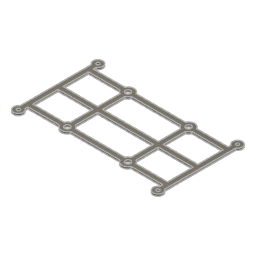
fc_vibration_dumper_DJI_F450 (Autodesk Fusion 360 design; units mm, degrees)
Autodesk Fusion 360 part; units mm, degrees
sketch "Sketch1" plane through (0, 0, 0) normal (0, 1, 0) x (1, 0, 0) in component "vibration_dumper_part_1"
  line L0 (0, 0) -> (62.5, 0)
  line L1 (62.5, 0) -> (62.5, -39.5)
  line L2 (62.5, -39.5) -> (0, -39.5)
  line L3 (0, -39.5) -> (0, 0)
  circle A0 centre (0, 0) radius 1.6
  circle A1 centre (62.5, 0) radius 1.6
  circle A2 centre (62.5, -39.5) radius 1.6
  circle A3 centre (0, -39.5) radius 1.6
  line L4 (0, -39.5) -> (0, -37)
  line L5 (62.5, -39.5) -> (62.5, -41.1)
  line L6 (62.5, -39.5) -> (62.5, -42)
  line L7 (0, -37) -> (62.5, -37)
  line L8 (62.5, -37) -> (62.5, -42)
  line L9 (62.5, -42) -> (0, -42)
  line L10 (0, -42) -> (0, -37)
  line L11 (0, -39.5) -> (2.5, -39.5)
  line L12 (0, 0) -> (-2.5, 0)
  line L13 (-2.5, 0) -> (2.5, 0)
  line L14 (2.5, 0) -> (2.5, -39.5)
  line L15 (2.5, -39.5) -> (-2.5, -39.5)
  line L16 (-2.5, -39.5) -> (-2.5, 0)
  line L17 (62.5, 0) -> (62.5, 2.5)
  line L18 (62.5, 2.5) -> (0, 2.5)
  line L19 (0, 2.5) -> (0, -2.5)
  line L20 (0, -2.5) -> (62.5, -2.5)
  line L21 (62.5, -2.5) -> (62.5, 2.5)
  line L22 (62.5, -39.5) -> (65, -39.5)
  line L23 (65, -39.5) -> (60, -39.5)
  line L24 (60, -39.5) -> (60, 0)
  line L25 (60, 0) -> (65, 0)
  line L26 (65, 0) -> (65, -39.5)
  circle A4 centre (0, 0) radius 5
  circle A5 centre (62.5, 0) radius 5
  circle A6 centre (0, -39.5) radius 5
  circle A7 centre (62.5, -39.5) radius 5
  line L27 (0, -39.5) -> (0, -51)
  line L28 (0, 0) -> (0, 11.5)
  line L29 (0, 11.5) -> (62.5, 11.5)
  line L30 (62.5, 11.5) -> (62.5, -51)
  line L31 (62.5, -51) -> (0, -51)
  line L32 (0, -51) -> (0, 11.5)
  circle A8 centre (0, 11.5) radius 2.75
  circle A9 centre (62.5, 11.5) radius 2.75
  circle A10 centre (0, -51) radius 2.75
  circle A11 centre (62.5, -51) radius 2.75
  circle A12 centre (0, 11.5) radius 6.25
  circle A13 centre (0, -51) radius 6.25
  circle A14 centre (62.5, -51) radius 6.25
  circle A15 centre (62.5, 11.5) radius 6.25
  line L33 (60, 0) -> (65, 0)
  line L34 (65, 0) -> (65, 7)
  line L35 (65, 7) -> (60, 7)
  line L36 (60, 7) -> (60, 0)
  line L37 (-2.5, 0) -> (2.5, 0)
  line L38 (2.5, 0) -> (2.5, 7)
  line L39 (2.5, 7) -> (-2.5, 7)
  line L40 (-2.5, 7) -> (-2.5, 0)
  line L41 (-2.5, -39.5) -> (2.5, -39.5)
  line L42 (2.5, -39.5) -> (2.5, -46.5)
  line L43 (2.5, -46.5) -> (-2.5, -46.5)
  line L44 (-2.5, -46.5) -> (-2.5, -39.5)
  line L45 (60, -39.5) -> (65, -39.5)
  line L46 (65, -39.5) -> (65, -46.5)
  line L47 (65, -46.5) -> (60, -46.5)
  line L48 (60, -46.5) -> (60, -39.5)
  dimension "d1" = 62.5
  dimension "d2" = 39.5
  dimension "d3" = 3.2
  dimension "d4" = 3.2
  dimension "d5" = 3.2
  dimension "d6" = 3.2
  dimension "d7" = 2.5
  dimension "d8" = 2.5
  dimension "d9" = 2.5
  dimension "d10" = 5
  dimension "d11" = 5
  dimension "d12" = 10
  dimension "d13" = 10
  dimension "d14" = 10
  dimension "d15" = 10
  dimension "d18" = 11.5
  dimension "d19" = 11.5
  dimension "d20" = 62.5
  dimension "d21" = 5.5
  dimension "d22" = 5.5
  dimension "d23" = 5.5
  dimension "d24" = 5.5
  dimension "d25" = 12.5
  dimension "d26" = 12.5
  dimension "d27" = 12.5
  dimension "d28" = 12.5
  dimension "d29" = 7
  dimension "d30" = 7
  dimension "d31" = 7
  constraint horizontal L0
  constraint vertical L1
  constraint horizontal L2
  constraint vertical L3
  constraint coincident L0.start L3.end
  constraint coincident L0.end L1.start
  constraint coincident L1.end L2.start
  constraint coincident L2.end L3.start
  constraint perpendicular L2 L4
  constraint coincident A2 L5.end
  constraint perpendicular L2 L5
  constraint parallel L5 L6
  constraint horizontal L7
  constraint vertical L8
  constraint horizontal L9
  constraint vertical L10
  constraint perpendicular L4 L11
  constraint perpendicular L3 L12
  constraint horizontal L13
  constraint vertical L14
  constraint horizontal L15
  constraint vertical L16
  constraint perpendicular L0 L17
  constraint horizontal L18
  constraint vertical L19
  constraint horizontal L20
  constraint vertical L21
  constraint coincident L3 L19.end
  constraint perpendicular L5 L22
  constraint horizontal L23
  constraint vertical L24
  constraint horizontal L25
  constraint vertical L26
  constraint coincident L0 L24.end
  constraint concentric A1 A5
  constraint concentric A3 A6
  constraint perpendicular L15 L27
  constraint perpendicular L0 L28
  constraint horizontal L29
  constraint vertical L30
  constraint horizontal L31
  constraint vertical L32
  constraint coincident L28.end L29.start
  constraint coincident L29.end L30.start
  constraint coincident L27.end L31.end
  constraint coincident L30.end L31.start
  constraint concentric A8 A12
  constraint concentric A11 A14
  constraint concentric A9 A15
  constraint horizontal L33
  constraint vertical L34
  constraint horizontal L35
  constraint vertical L36
  constraint horizontal L37
  constraint vertical L38
  constraint horizontal L39
  constraint vertical L40
  constraint horizontal L41
  constraint vertical L42
  constraint horizontal L43
  constraint vertical L44
  constraint horizontal L45
  constraint vertical L46
  constraint horizontal L47
  constraint vertical L48
  measures "d1" distance of L0.start L0.end
  measures "d2" distance of L0.start L2.end
  measures "d3" diameter of A0
  measures "d4" diameter of A1
  measures "d5" diameter of A2
  measures "d6" diameter of A3
  measures "d7" distance of L2.end L4.end
  measures "d8" distance of L1.end L6.end
  measures "d9" distance of L2.end L11.end
  measures "d10" distance of L17.end L20.end
  measures "d11" distance of L22.end L23.end
  measures "d12" diameter of A4
  measures "d13" diameter of A5
  measures "d14" diameter of A6
  measures "d15" diameter of A7
  measures "d18" distance of L2.end L27.end
  measures "d19" distance of L0.start L28.end
  measures "d20" distance of L28.end L27.end
  measures "d21" diameter of A8
  measures "d22" diameter of A9
  measures "d23" diameter of A10
  measures "d24" diameter of A11
  measures "d25" diameter of A12
  measures "d26" diameter of A13
  measures "d27" diameter of A14
  measures "d28" diameter of A15
  measures "d29" distance of L12.end L39.end
  measures "d30" distance of L15.end L43.end
  measures "d31" distance of L23.end L47.end
extrude "Extrude1" add sketch "Sketch1" along normal blind 2 contours L0 A0 L13 L18 L19 L28 L32 L37 L38 | L0 L3 A0 L13 L14 L19 L20 L32 L37 | L3 A0 L12 L13 L16 L19 A4 L32 L37 | A0 L12 L13 L19 A4 L28 L32 L37 L40 | L0 L18 A4 L38 | L0 L14 L20 A4 | L3 L14 L20 A4 L32 | L16 A4 L40 | L18 A4 L28 L32 L38 | L0 L18 A4 A5 | L0 L20 A4 A5 | L14 L20 A4 | L18 A4 L38 | L3 L14 A4 A6 L32 | L3 L16 A4 A6 L32 | L0 L18 A5 L36 | L0 L20 L24 A5 | L3 L7 L14 A6 L32 | L3 A3 L4 L10 L15 L16 A6 L32 L41 | L16 A6 L44 | L0 A1 L17 L18 L21 L25 L30 L33 L36 | L0 L1 A1 L20 L21 L24 L25 L30 L33 | L18 A5 L36 | L20 L24 A5 | L7 L14 A6 | L2 L3 A3 L4 L7 L10 L11 L14 L15 L32 L41 | A3 L10 L15 A6 L27 L32 L41 L44 | L1 L20 L24 A5 L30 | L18 A5 L30 L36 | L1 L24 A5 A7 L30 | L2 L7 L14 A6 | L2 L7 A6 A7 | L9 A6 L27 L32 L42 | A1 L17 L21 L25 A5 L30 L33 L34 | L1 A1 L21 L25 L26 A5 L30 L33 | L1 L7 L24 A7 L30 | L7 L24 A7 | L1 L26 A5 A7 L30 | L2 A3 L9 L10 L11 L15 L27 L32 L41 L42 | L2 L9 A6 L42 | L2 L7 L24 A7 | L2 L9 A6 A7 | L9 A6 L42 | L26 A5 L34 | L1 L2 A2 L7 L8 L23 L24 L30 L45 | L1 A2 L8 L22 L23 L26 A7 L30 L45 | L2 L9 A7 L48 | L2 A2 L6 L8 L9 L23 L30 L45 L48 | L26 A7 L46 | L9 A7 L48 | L9 A7 L30 L48 | A2 L6 L8 L22 L23 A7 L30 L45 L46 makes body 1 in component "vibration_dumper_part_1"
extrude "Extrude2" add sketch "Sketch1" along normal blind 2 contours A4 L28 L32 A12 L40 | A4 L28 L32 A12 L38 | L28 L32 A12 L39 L40 | L28 L29 L32 A8 A12 L39 L40 | L28 L32 A12 L38 L39 | L28 L29 L32 A8 A12 L38 L39 | A6 L27 L32 A13 L44 | A5 L30 A15 L36 | A6 L27 L32 A13 L42 | L27 L31 L32 A10 A13 L43 L44 | L27 L32 A13 L43 L44 | L29 L30 A9 A15 L34 L35 | L29 L30 A9 A15 L35 L36 | A5 L30 A15 L34 | L30 A15 L35 L36 | L27 L32 A13 L42 L43 | L27 L31 L32 A10 A13 L42 L43 | L30 A15 L34 L35 | L30 L31 A11 A14 L47 L48 | L30 L31 A11 A14 L46 L47 | A7 L30 A14 L48 | L30 A14 L47 L48 | L30 A14 L46 L47 | A7 L30 A14 L46 bodies 1 in component "vibration_dumper_part_1"
sketch "Sketch2" plane through (0, 0, 0) normal (0, 1, 0) x (1, 0, 0) in component "vibration_dumper_part_1"
  circle A0 centre (62.5, 11.5) radius 2.75
  circle A1 centre (62.5, 11.5) radius 6.25
  circle A2 centre (0, 11.5) radius 2.75
  circle A3 centre (0, 11.5) radius 6.25
  circle A4 centre (0, -51) radius 2.75
  circle A5 centre (0, -51) radius 6.25
  circle A6 centre (62.5, -51) radius 2.6926
  circle A7 centre (62.5, -51) radius 6.25
  line L0 (65, -46.5) -> (60, -46.5)
  line L1 (60, -46.5) -> (60, 7)
  line L2 (60, 7) -> (65, 7)
  line L3 (65, 7) -> (65, -46.5)
  line L4 (2.5, -46.5) -> (-2.5, -46.5)
  line L5 (-2.5, -46.5) -> (-2.5, 7)
  line L6 (-2.5, 7) -> (2.5, 7)
  line L7 (2.5, 7) -> (2.5, -46.5)
  line L8 (62.5, 11.5) -> (62.5, -51)
  line L9 (62.5, -51) -> (62.5, -48.5)
  line L10 (0, 11.5) -> (62.5, 11.5)
  line L11 (62.5, 11.5) -> (62.5, 9)
  line L12 (62.5, 9) -> (0, 9)
  line L13 (0, 9) -> (0, 14)
  line L14 (0, 14) -> (62.5, 14)
  line L15 (62.5, 14) -> (62.5, 9)
  line L16 (62.5, -48.5) -> (0, -48.5)
  line L17 (0, -48.5) -> (0, -53.5)
  line L18 (0, -53.5) -> (62.5, -53.5)
  line L19 (62.5, -53.5) -> (62.5, -48.5)
  point P0 (62.5, 11.5)
  point P1 (0, 11.5)
  point P2 (0, -51)
  point P3 (62.5, -51)
  point P4 (65, -46.5)
  point P5 (60, 7)
  point P6 (2.5, -46.5)
  point P7 (-2.5, 7)
  dimension "d34" = 2.5
  dimension "d35" = 2.5
  dimension "d36" = 5
  dimension "d37" = 5
  constraint coincident P0 A0.centre
  constraint coincident P1 A2.centre
  constraint coincident P2 A4.centre
  constraint coincident P3 A6.centre
  constraint horizontal L0
  constraint vertical L1
  constraint horizontal L2
  constraint vertical L3
  constraint coincident P5 L1.end
  constraint coincident P4 L0.start
  constraint horizontal L4
  constraint vertical L5
  constraint horizontal L6
  constraint vertical L7
  constraint coincident P7 L5.end
  constraint coincident P6 L4.start
  constraint parallel L8 L9
  constraint perpendicular L10 L11
  constraint horizontal L12
  constraint vertical L13
  constraint horizontal L14
  constraint vertical L15
  constraint horizontal L16
  constraint vertical L17
  constraint horizontal L18
  constraint vertical L19
  measures "d34" distance of P3 L9.end
  measures "d35" distance of P0 L11.end
  measures "d36" distance of L11.end L14.end
  measures "d37" distance of L9.end L18.end
extrude "Extrude3" add sketch "Sketch2" along normal blind 2 separate body contours A0 A1 L2 L3 L8 L14 | A0 A1 L10 L14 | A0 A1 L1 L2 L8 L12 | A0 A1 L10 L12 | A1 A3 L10 L14 | A1 L1 L2 L8 | A1 L2 L3 L8 | A1 A3 L10 L12 | A2 A3 L5 L6 L7 L12 L14 | A2 A3 L10 L14 | A1 A7 L1 L8 | A1 A7 L3 L8 | A2 A3 L10 L12 | A3 L5 L6 L7 | A3 A5 L5 L7 | A7 L0 L1 L8 | A7 L0 L3 L8 | A6 A7 L0 L3 L8 L18 | A4 A5 L4 L5 L7 L16 L18 | A5 L4 L5 L7 | A6 A7 L0 L1 L8 L16 | A4 A5 L16 L18 | A5 A7 L16 L18 | A6 A7 L16 L18 makes body 2 in component "vibration_dumper_part_1"
sketch "Sketch3" plane through (0, 0, 0) normal (0, 1, 0) x (1, 0, 0) in component "vibration_dumper_part_1"
  line L0 (0, -48.5) -> (0, -53.5)
  line L1 (0, -51) -> (-43.75, -51)
  line L2 (62.5, -53.5) -> (62.5, -48.5)
  line L3 (62.5, -51) -> (106.25, -51)
  line L4 (106.25, -51) -> (103.25, -51)
  line L5 (-43.75, -51) -> (-40.75, -51)
  line L6 (103.25, 11.5) -> (-40.75, 11.5)
  line L7 (62.5, -51) -> (62.5, -64.75)
  line L8 (62.5, 11.5) -> (62.5, 25.25)
  line L9 (62.5, -64.75) -> (62.5, -60.75)
  line L10 (62.5, 25.25) -> (62.5, 21.25)
  line L11 (62.5, 21.25) -> (103.25, 21.25)
  line L12 (103.25, 21.25) -> (103.25, 11.5)
  line L13 (103.25, 11.5) -> (62.5, 11.5)
  line L14 (62.5, 11.5) -> (62.5, 21.25)
  line L15 (103.25, -51) -> (62.5, -51)
  line L16 (62.5, -51) -> (62.5, -60.75)
  line L17 (62.5, -60.75) -> (103.25, -60.75)
  line L18 (103.25, -60.75) -> (103.25, -51)
  line L19 (0, -51) -> (-40.75, -51)
  line L20 (-40.75, -51) -> (-40.75, -60.75)
  line L21 (-40.75, -60.75) -> (0, -60.75)
  line L22 (0, -60.75) -> (0, -51)
  line L23 (0, 11.5) -> (-40.75, 11.5)
  line L24 (-40.75, 11.5) -> (-40.75, 21.25)
  line L25 (-40.75, 21.25) -> (0, 21.25)
  line L26 (0, 21.25) -> (0, 11.5)
  circle A0 centre (103.25, -60.75) radius 1.6
  circle A1 centre (103.25, -60.75) radius 5
  circle A2 centre (-40.75, -60.75) radius 1.6
  circle A3 centre (-40.75, -60.75) radius 5
  circle A4 centre (-40.75, 21.25) radius 1.6
  circle A5 centre (-40.75, 21.25) radius 5
  circle A6 centre (103.25, 21.25) radius 1.6
  circle A7 centre (103.25, 21.25) radius 5
  line L27 (103.25, -60.75) -> (105.75, -60.75)
  line L28 (105.75, -60.75) -> (100.75, -60.75)
  line L29 (100.75, -60.75) -> (100.75, 21.25)
  line L30 (100.75, 21.25) -> (105.75, 21.25)
  line L31 (105.75, 21.25) -> (105.75, -60.75)
  line L32 (-40.75, -60.75) -> (-43.25, -60.75)
  line L33 (-43.25, -60.75) -> (-38.25, -60.75)
  line L34 (-38.25, -60.75) -> (-38.25, 21.25)
  line L35 (-38.25, 21.25) -> (-43.25, 21.25)
  line L36 (-43.25, 21.25) -> (-43.25, -60.75)
  line L37 (0, 9) -> (-38.25, 9)
  line L38 (-38.25, 9) -> (-38.25, 14)
  line L39 (-38.25, 14) -> (0, 14)
  line L40 (0, 14) -> (0, 9)
  line L41 (62.5, 14) -> (100.75, 14)
  line L42 (100.75, 14) -> (100.75, 9)
  line L43 (100.75, 9) -> (62.5, 9)
  line L44 (62.5, 9) -> (62.5, 14)
  line L45 (62.5, -48.5) -> (100.75, -48.5)
  line L46 (100.75, -48.5) -> (100.75, -53.5)
  line L47 (100.75, -53.5) -> (62.5, -53.5)
  line L48 (62.5, -53.5) -> (62.5, -48.5)
  line L49 (0, -53.5) -> (-38.25, -53.5)
  line L50 (-38.25, -53.5) -> (-38.25, -48.5)
  line L51 (-38.25, -48.5) -> (0, -48.5)
  line L52 (0, -48.5) -> (0, -53.5)
  line L53 (100.75, -19.75) -> (-38.25, -19.75)
  line L54 (100.75, -19.75) -> (-38.25, -19.75)
  line L55 (-38.25, -19.75) -> (-38.25, -22.25)
  line L56 (-38.25, -22.25) -> (100.75, -22.25)
  line L57 (100.75, -22.25) -> (100.75, -19.75)
  line L58 (100.75, -19.75) -> (-38.25, -19.75)
  line L59 (-38.25, -19.75) -> (-38.25, -17.25)
  line L60 (-38.25, -17.25) -> (100.75, -17.25)
  line L61 (100.75, -17.25) -> (100.75, -19.75)
  point P0 (0, -51)
  point P1 (62.5, -51)
  point P2 (62.5, 11.5)
  point P3 (0, 11.5)
  point P4 (0, 9)
  point P5 (62.5, 14)
  dimension "d40" = 43.75
  dimension "d41" = 43.75
  dimension "d42" = 3
  dimension "d43" = 3
  dimension "d44" = 13.75
  dimension "d45" = 13.75
  dimension "d46" = 4
  dimension "d47" = 4
  dimension "d48" = 3.2
  dimension "d49" = 10
  dimension "d50" = 3.2
  dimension "d51" = 10
  dimension "d52" = 3.2
  dimension "d53" = 10
  dimension "d54" = 3.2
  dimension "d55" = 10
  dimension "d58" = 2.5
  dimension "d59" = 5
  dimension "d60" = 2.5
  dimension "d61" = 5
  dimension "d62" = 5
  dimension "d63" = 5
  dimension "d74" = 2.5
  dimension "d75" = 2.5
  constraint coincident P0 L1.start
  constraint perpendicular L0 L1
  constraint coincident P1 L3.start
  constraint perpendicular L2 L3
  constraint parallel L3 L4
  constraint parallel L1 L5
  constraint parallel L1 L6
  constraint perpendicular L3 L7
  constraint coincident P2 L8.start
  constraint perpendicular L6 L8
  constraint parallel L7 L9
  constraint parallel L8 L10
  constraint horizontal L11
  constraint vertical L12
  constraint horizontal L13
  constraint vertical L14
  constraint horizontal L15
  constraint vertical L16
  constraint horizontal L17
  constraint vertical L18
  constraint horizontal L19
  constraint vertical L20
  constraint horizontal L21
  constraint vertical L22
  constraint horizontal L23
  constraint vertical L24
  constraint horizontal L25
  constraint vertical L26
  constraint coincident P3 L23.start
  constraint coincident L17.end L18.start
  constraint concentric A0 A1
  constraint coincident L20.end L21.start
  constraint coincident L24.end L25.start
  constraint concentric A4 A5
  constraint coincident L11.end L12.start
  constraint concentric A6 A7
  constraint perpendicular L18 L27
  constraint horizontal L28
  constraint vertical L29
  constraint horizontal L30
  constraint vertical L31
  constraint perpendicular L20 L32
  constraint horizontal L33
  constraint vertical L34
  constraint horizontal L35
  constraint vertical L36
  constraint coincident L25 L34.end
  constraint horizontal L37
  constraint vertical L38
  constraint horizontal L39
  constraint vertical L40
  constraint coincident L34 L38.end
  constraint coincident P4 L37.start
  constraint horizontal L41
  constraint vertical L42
  constraint horizontal L43
  constraint vertical L44
  constraint coincident L29 L42.end
  constraint coincident P5 L41.start
  constraint horizontal L45
  constraint vertical L46
  constraint horizontal L47
  constraint vertical L48
  constraint coincident L29 L46.end
  constraint coincident L2.end L45.start
  constraint horizontal L49
  constraint vertical L50
  constraint horizontal L51
  constraint vertical L52
  constraint coincident L34 L50.end
  constraint coincident L0.end L49.start
  constraint midpoint L29 L53.start
  constraint midpoint L34 L53.end
  constraint horizontal L54
  constraint vertical L55
  constraint horizontal L56
  constraint vertical L57
  constraint horizontal L58
  constraint vertical L59
  constraint horizontal L60
  constraint vertical L61
  measures "d40" distance of P0 L1.end
  measures "d41" distance of P1 L3.end
  measures "d42" distance of L3.end L4.end
  measures "d43" distance of L1.end L5.end
  measures "d44" distance of P1 L7.end
  measures "d45" distance of P2 L8.end
  measures "d46" distance of L7.end L9.end
  measures "d47" distance of L8.end L10.end
  measures "d48" diameter of A0
  measures "d49" diameter of A1
  measures "d50" diameter of A2
  measures "d51" diameter of A3
  measures "d52" diameter of A4
  measures "d53" diameter of A5
  measures "d54" diameter of A6
  measures "d55" diameter of A7
  measures "d58" distance of L17.end L27.end
  measures "d59" distance of L27.end L28.end
  measures "d60" distance of L20.end L32.end
  measures "d61" distance of L32.end L33.end
  measures "d62" distance of P4 L39.end
  measures "d63" distance of L2.end L2.start
  measures "d74" distance of L53.start L56.end
  measures "d75" distance of L53.start L60.end
extrude "Extrude4" add sketch "Sketch3" along normal blind 2 separate body contours L21 A2 A3 L32 L33 L36 | L21 A3 L34 | L20 L21 A2 A3 L33 L34 | L20 A2 A3 L32 L33 L36 | L24 A4 A5 L35 L36 | L25 A4 A5 L35 L36 | L25 A5 L34 | L24 L25 A4 A5 L34 L35 | L18 A0 A1 L27 L28 L31 | L17 L18 A0 A1 L28 L29 | L17 A1 L29 | L11 A6 A7 L30 L31 | L12 A6 A7 L30 L31 | L17 A0 A1 L27 L28 L31 | L11 L12 A6 A7 L29 L30 | L11 A7 L29 makes body 3 at (107.0981, 0, -21.0016) makes body 4 at (-36.9079, 0, -20.9221) makes body 5 at (107.0981, 0, 60.9984) makes body 6 at (-36.9079, 0, 61.0779) in component "vibration_dumper_part_1"
extrude "Extrude5" cut sketch "Sketch3" along normal blind 2 contours L1 L5 L6 L19 L23 L24 A5 L34 L36 L38 L50 L55 L59 | L1 L19 L20 A3 L34 L50 | L1 L5 L20 A3 L36 | L3 L4 L6 L12 L13 L15 A7 L29 L31 L42 L46 L57 L61 | L2 L3 L15 L29 L45 L46 L48 | L6 L23 L34 L37 L38 L40 | L2 L3 L7 L15 L16 L29 L46 L47 L48 | L3 L15 L18 A1 L29 L46 | L6 L23 L24 A5 L34 L38 | L6 L23 L26 L34 L38 L39 L40 | L6 L13 L29 L42 L43 L44 | L3 L4 L18 A1 L31 | L6 L12 L13 A7 L29 L42 | L6 L8 L13 L14 L29 L41 L42 L44 bodies 2 in component "vibration_dumper_part_1"
extrude "Extrude6" cut sketch "Sketch3" along normal blind 2 contours L0 L1 L19 L34 L50 L51 L52 | L0 L1 L19 L22 L34 L49 L50 L52 bodies 2 in component "vibration_dumper_part_1"
extrude "Extrude7" add sketch "Sketch3" along normal blind 2 contours L0 L1 L19 L34 L50 L51 L52 | L0 L1 L19 L22 L34 L49 L50 L52 | L1 L5 L6 L19 L23 L24 A5 L34 L36 L38 L50 L55 L59 | L1 L19 L20 A3 L34 L50 | L1 L5 L20 A3 L36 | L3 L4 L6 L12 L13 L15 A7 L29 L31 L42 L46 L57 L61 | L2 L3 L15 L29 L45 L46 L48 | L6 L23 L34 L37 L38 L40 | L2 L3 L7 L15 L16 L29 L46 L47 L48 | L3 L15 L18 A1 L29 L46 | L6 L23 L24 A5 L34 L38 | L6 L23 L26 L34 L38 L39 L40 | L6 L13 L29 L42 L43 L44 | L3 L4 L18 A1 L31 | L6 L12 L13 A7 L29 L42 | L6 L8 L13 L14 L29 L41 L42 L44 bodies 2 3 4 5 6 in component "vibration_dumper_part_1"
extrude "Extrude8" cut sketch "Sketch2" along normal blind 14 contours A0 L8 L11 L14 L15 | A2 L12 L13 L14 | A6 L8 L9 L18 L19 | A4 L16 L17 L18 picked at (-0.9142, -50.9321) bodies 2 in component "vibration_dumper_part_1"
extrude "Extrude9" add sketch "Sketch3" along normal blind 2 separate body contours L11 A6 A7 L30 L31 | L12 A6 A7 L30 L31 | L11 L12 A6 A7 L29 L30 | L11 A7 L29 makes body 7 in component "vibration_dumper_part_1"
extrude "Extrude10" add sketch "Sketch3" along normal blind 2 separate body contours L29 L34 L53 L54 L55 L56 L57 L58 | L29 L34 L53 L54 L58 L59 L60 L61 makes body 8 in component "vibration_dumper_part_1"
combine "Combine1" operation add target body 8 tool bodies 2 in component "vibration_dumper_part_1"
component "vibration_dumper_part_1" placed x (1, 0, 0) y (0, 1, 0) z (0, 0, 1) at (0, 0, 0)
hidden bodies 1 7
